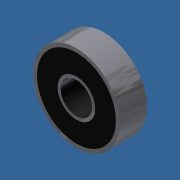
# Autodesk Inventor part: SM-M07
Saved by Autodesk Inventor 2012 SP1 (Build 160190100, 190)
## iProperties
Created: 2011-09-26
Part Number: SM-M07
Document SubType Name: Modeling
Designer: ERF
Density: 1 g/cm^3
Description: Standard 608-2RS Skateboard Bearing
Material: Default
Stock Number: skate_bearing
Vendor: McMasterCarr
Project: Shapeoko
Mass: 2.30662 g
Surface Area: 13.204 cm^2
Volume: 2.30662 cm^3
Title: Z-Axis Bearing
Author: ERF
Autodesk Inventor part; units mm, degrees
ref_plane "YZ Plane" through (0, 0, 0) normal (1, 0, 0) x (0, 1, 0)
ref_plane "XZ Plane" through (0, 0, 0) normal (0, 1, 0) x (-1, 0, 0)
ref_plane "XY Plane" through (0, 0, 0) normal (0, 0, 1) x (1, 0, 0)
sketch "Sketch1" plane through (0, 0, 0) normal (0, 0, 1) x (1, 0, 0)
  circle A0 centre (0, 0) radius 4
  circle A1 centre (0, 0) radius 11
  dimension "d0" = 8
  dimension "d1" = 22
  constraints: 2 centre point, 1 coincident
  measures "d0" diameter of A0
  measures "d1" diameter of A1
extrude "Extrusion1" add sketch "Sketch1" along normal blind 7
sketch "Sketch2" plane through (0, 0, 7) normal (0, 0, 1) x (1, 0, 0)
  circle A0 centre (0, 0) radius 11 projected
  circle A1 centre (0, 0) radius 10.0393
  circle A2 centre (0, 0) radius 4.7793
  constraints: 2 centre point, 2 coincident
extrude "Extrusion2" cut sketch "Sketch2" against normal blind 0.01 contours A1
body "Solid1"
